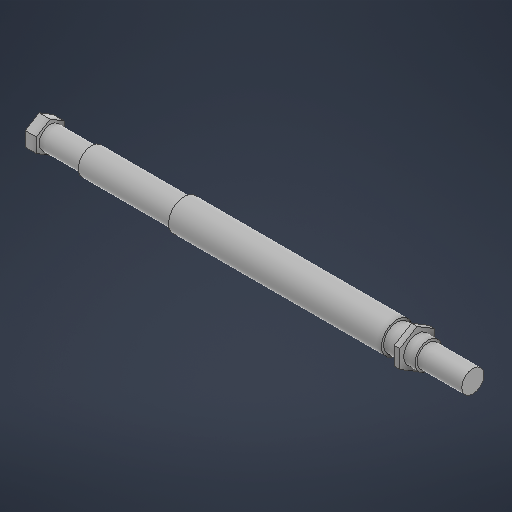
# Autodesk Inventor part: Welle
Saved by Autodesk Inventor 2026 (Build 300175050, 175E)
## iProperties
Created: 2025-11-20
Part Number: Welle
Material: Generisch
Document SubType Name: Modeling
Designer: aurich
Density: 1 g/cm^3
Appearance: Vorgabe
Author: aurich
Autodesk Inventor part; units mm, degrees
ref_plane "YZ Plane" through (0, 0, 0) normal (1, 0, 0) x (0, 1, 0)
ref_plane "XZ Plane" through (0, 0, 0) normal (0, 1, 0) x (-1, 0, 0)
ref_plane "XY Plane" through (0, 0, 0) normal (0, 0, 1) x (1, 0, 0)
ref_plane "Arbeitsebene1" through (62.6214, -145.6709, 60.7697) normal (-1, 0, 0) x (0, -0.0041874, 0.9999912)
sketch "Skizze1" plane through (62.6214, -145.6709, 60.7697) normal (-1, 0, 0) x (0, -0.0041874, 0.9999912)
  circle A0 centre (0, 0) radius 10
  point P0 (-61.3791, 145.4152)
  dimension "d0" = 20
  constraints: 1 centre point
  measures "d0" diameter of A0
extrude "Extrusion1" add sketch "Skizze1" against normal blind 37
sketch "Skizze2" plane through (99.6214, -145.6709, 60.7697) normal (1, 0, 0) x (0, 0, -1)
  circle A0 centre (0, 0) radius 10 projected
  circle A1 centre (0, 0) radius 12
  point P0 (60.7697, 145.6709)
  dimension "d3" = 24
  constraints: 1 centre point, 1 coincident
  measures "d3" diameter of A1
extrude "Extrusion2" add sketch "Skizze2" along normal blind 83 contours A0 | A1
sketch "Skizze3" plane through (182.6214, -145.6709, 60.7697) normal (1, 0, 0) x (0, 0, -1)
  circle A0 centre (0, 0) radius 12 projected
  circle A1 centre (0, 0) radius 14
  point P0 (60.7697, 145.6709)
  dimension "d6" = 28
  constraints: 1 centre point, 1 coincident
  measures "d6" diameter of A1
extrude "Extrusion3" add sketch "Skizze3" along normal blind 191 contours A0 | A1
sketch "Skizze4" plane through (373.6214, -145.6709, 60.7697) normal (1, 0, 0) x (0, 0, -1)
  circle A0 centre (0, 0) radius 10 projected
  circle A1 centre (0, 0) radius 12
  point P0 (60.7697, 145.6709)
  dimension "d9" = 24
  constraints: 1 centre point, 1 coincident
  measures "d9" diameter of A1
extrude "Extrusion4" add sketch "Skizze4" along normal blind 13 contours A0 | A1
sketch "Skizze5" plane through (386.6214, -145.6709, 60.7697) normal (1, 0, 0) x (0, 0, -1)
  circle A0 centre (0, 0) radius 12 projected
  circle A1 centre (0, 0) radius 17.5 construction
  line L0 (-8.1188, 15.5028) -> (8.1188, 15.5028)
  line L1 (8.1188, 15.5028) -> (17.5, 0)
  line L2 (17.5, 0) -> (8.1188, -15.5028)
  line L3 (8.1188, -15.5028) -> (-8.1188, -15.5028)
  line L4 (-8.1188, -15.5028) -> (-17.5, 0)
  line L5 (-17.5, 0) -> (-8.1188, 15.5028)
  point P0 (60.7697, 145.6709)
  dimension "d12" = 35
  constraints: 12 end point, 6 point on circle, 2 parallel, 2 vertical alignment, 1 centre point, 1 coincident, 1 horizontal
  measures "d12" diameter of A1
extrude "Extrusion5" add sketch "Skizze5" along normal blind 5 contours A0 | L0 L1 L2 L3 L4 L5
sketch "Skizze6" plane through (391.6214, -145.6709, 60.7697) normal (1, 0, 0) x (0, 0, -1)
  circle A0 centre (0, 0) radius 10 projected
  circle A1 centre (0, 0) radius 12
  point P0 (60.7697, 145.6709)
  dimension "d15" = 24
  constraints: 1 centre point, 1 coincident
  measures "d15" diameter of A1
extrude "Extrusion6" add sketch "Skizze6" along normal blind 10 contours A0 | A1
sketch "Skizze7" plane through (401.6214, -145.6709, 60.7697) normal (1, 0, 0) x (0, 0, -1)
  circle A0 centre (0, 0) radius 10 projected
  circle A1 centre (0, 0) radius 10
  point P0 (60.7697, 145.6709)
  dimension "d18" = 20
  constraints: 1 centre point, 1 coincident
  measures "d18" diameter of A1
extrude "Extrusion7" add sketch "Skizze7" along normal blind 40
sketch "Skizze8" plane through (62.6214, -145.6709, 60.7697) normal (-1, 0, 0) x (0, 0, 1)
  line L0 (8.1188, 15.5028) -> (17.5, 0) projected
  line L1 (17.5, 0) -> (8.1188, -15.5028) projected
  line L2 (-8.1188, 15.5028) -> (8.1188, 15.5028) projected
  line L3 (-17.5, 0) -> (-8.1188, 15.5028) projected
  line L4 (-8.1188, -15.5028) -> (-17.5, 0) projected
  line L5 (8.1188, -15.5028) -> (-8.1188, -15.5028) projected
  line L6 (13.9935, 0) -> (6.4276, 12.5028)
  line L7 (6.4276, 12.5028) -> (-6.4276, 12.5028)
  line L8 (-6.4276, 12.5028) -> (-13.9935, 0)
  line L9 (-13.9935, 0) -> (-6.4276, -12.5028)
  line L10 (-6.4276, -12.5028) -> (6.4276, -12.5028)
  line L11 (6.4276, -12.5028) -> (13.9935, 0)
  point P0 (-60.7697, 145.6709)
  dimension "d23" = 3
  constraints: 12 end point, 5 other
  measures "d23" distance between parallel lines of L0 L6
extrude "Extrusion8" add sketch "Skizze8" along normal blind 10 contours L11 L10 L9 L8 L7 L6
